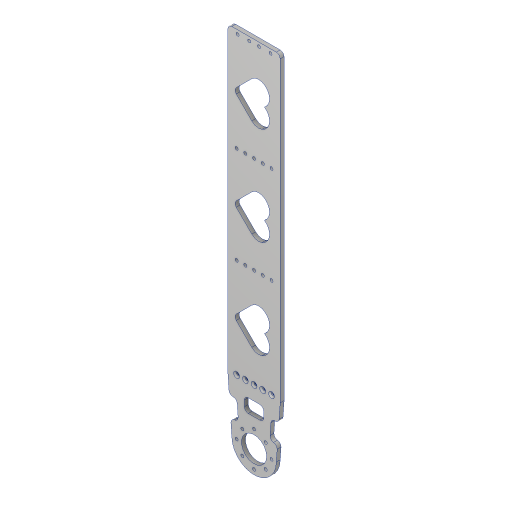
# Autodesk Inventor part: J2L1_H_Side2
Saved by Autodesk Inventor 2023.2 (Build 272271000, 271)
## iProperties
Created: 2021-07-07
Part Number: J2L1_H_Side2
Material: 알루미늄 6061
Document SubType Name: Modeling
Designer: user
Density: 2.7 g/cm^3
Appearance: 알루미늄 - 평지
Mass: 220.087 g
Surface Area: 468.714 cm^2
Volume: 81.5136 cm^3
Author: user
Autodesk Inventor part; units mm, degrees
ref_plane "YZ Plane" through (0, 0, 0) normal (1, 0, 0) x (0, 1, 0)
ref_plane "XZ Plane" through (0, 0, 0) normal (0, 1, 0) x (-1, 0, 0)
ref_plane "XY Plane" through (0, 0, 0) normal (0, 0, 1) x (1, 0, 0)
sketch "스케치1" plane through (0, 0, 0) normal (0, 0, 1) x (1, 0, 0)
  circle A0 centre (0, 0) radius 13
  circle A1 centre (0, 0) radius 23
  line L0 (27, 0) -> (-27, 0)
  line L1 (-27, 0) -> (-27, 62)
  line L2 (-27, 62) -> (27, 62)
  line L3 (27, 62) -> (27, 0)
  line L4 (27, 62) -> (27, 55)
  line L5 (27, 62) -> (34, 62) construction
  line L6 (27, 55) -> (23, 0)
  line L7 (-27, 62) -> (-27, 55)
  line L8 (-27, 62) -> (-20, 62) construction
  line L9 (-27, 55) -> (-23, 0)
  dimension "d0" = 26
  dimension "d1" = 46
  dimension "d2" = 54
  dimension "d3" = 62
  dimension "d4" = 27
  dimension "d5" = 0
  dimension "d6" = 7
  dimension "d7" = 90
  dimension "d8" = 7
  dimension "d9" = 90
  constraints: 20 end point, 3 horizontal, 3 parallel, 3 perpendicular, 2 centre point, 2 coincident, 2 point on circle, 2 point on line, 1 collinear
  measures "d0" diameter of A0
  measures "d1" diameter of A1
  measures "d2" distance of L1.end L2.end
  measures "d3" distance of L0.end L1.end
  measures "d4" distance from line of L3 point (0, 0)
  measures "d5" distance from line of point (0, 0) L0
  measures "d6" distance of L2.end L4.end
  measures "d7" angle of L4 L5
  measures "d8" distance of L1.end L7.end
  measures "d9" angle of L7 L8
extrude "돌출1" add sketch "스케치1" along normal blind 4 contours L0 A0 | L0 A1 A0 | A0 L0 A1 | A0 L0 | A1 L9 L1 L2 L3 L6
sketch "스케치2" plane through (0, 0, 4) normal (0, 0, 1) x (1, 0, 0)
  circle A0 centre (0, 0) radius 13
  dimension "d12" = 26
  constraints: 1 centre point, 1 coincident
  measures "d12" diameter of A0
extrude "돌출2" cut sketch "스케치2" against normal up to surface (4 mm away)
sketch "스케치3" plane through (0, 0, 4) normal (0, 0, 1) x (1, 0, 0)
  line L0 (-0.15, -20.7995) -> (-0.15, -19.593)
  arc A0 (-0.15, -16.407) -> (-0.15, -19.593) centre (0, -18) ccw
  line L1 (-0.15, -16.407) -> (-0.15, -12.9991)
  arc A1 (0.15, -12.9991) -> (-0.15, -12.9991) centre (0, 0) ccw
  line L2 (0.15, -16.407) -> (0.15, -12.9991)
  arc A2 (0.15, -19.593) -> (0.15, -16.407) centre (0, -18) ccw
  line L3 (0.15, -20.7995) -> (0.15, -19.593)
  arc A3 (0.15, -20.7995) -> (-0.15, -20.7995) centre (0, 0) ccw
  circle A4 centre (12, 12) radius 1.6
  circle A5 centre (-18, 0) radius 1.6
  circle A6 centre (-12, 12) radius 1.6
  circle A7 centre (-12, -12) radius 1.6
  circle A8 centre (18, 0) radius 1.6
  circle A9 centre (12, -12) radius 1.6
  circle A10 centre (6, 18) radius 1
  circle A11 centre (-6, 18) radius 1
  circle A12 centre (-18, 6) radius 1
  circle A13 centre (-18, -6) radius 1
  circle A14 centre (-6, -18) radius 1
  circle A15 centre (6, -18) radius 1
  circle A16 centre (18, -6) radius 1
  circle A17 centre (18, 6) radius 1
  circle A18 centre (0, 18) radius 1.6
  circle A19 centre (0, 0) radius 12.5
  line L4 (-27, -21) -> (-21, -21)
  line L5 (-21, -21) -> (-21, -27)
  line L6 (25, -27) -> (27, -25)
  line L7 (27, -25) -> (27, 25)
  line L8 (27, 25) -> (25, 27)
  line L9 (25, 27) -> (-25, 27)
  line L10 (-25, 27) -> (-27, 25)
  line L11 (-27, 25) -> (-27, -25)
  line L12 (-27, -25) -> (-25, -27)
  line L13 (-25, -27) -> (25, -27)
  circle A20 centre (0, 0) radius 26.75
  circle A21 centre (24, -24) radius 1.6
  circle A22 centre (-24, -24) radius 1.6
  circle A23 centre (24, 24) radius 1.6
  circle A24 centre (-24, 24) radius 1.6
  circle A25 centre (0, -18) radius 1.6
  dimension "d15" = 3.2
  constraints: 28 end point, 26 centre point, 8 point on circle, 1 coincident
  measures "d15" diameter of A25
extrude "돌출3" cut sketch "스케치3" against normal up to surface (4 mm away) contours A0 A25 A2 | A4 | A5 | A6 | A7 | A8 | A9 | A18
sketch "스케치4" plane through (0, 0, 4) normal (0, 0, 1) x (1, 0, 0)
  circle A0 centre (0, 18) radius 1.6 projected
  circle A1 centre (12, 12) radius 1.6 projected
  circle A2 centre (-12, 12) radius 1.6 projected
  circle A3 centre (-18, 0) radius 1.6 projected
  circle A4 centre (12, -12) radius 1.6 projected
  circle A5 centre (0, -18) radius 1.6 projected
  circle A6 centre (-12, -12) radius 1.6 projected
  circle A7 centre (18, 0) radius 1.6 projected
  circle A8 centre (0, 0) radius 13 projected
  line L0 (27, 62) -> (-27, 62) projected
  line L1 (-27, 62) -> (-27, 55) projected
  line L2 (-27, 55) -> (-23, 0) projected
  arc A9 (-23, 0) -> (23, 0) centre (0, 0) ccw projected
  line L3 (23, 0) -> (27, 55) projected
  line L4 (27, 55) -> (27, 62) projected
  circle A10 centre (-18, 57.5) radius 1.6
  circle A11 centre (-9, 57.5) radius 1.6
  circle A12 centre (0, 57.5) radius 1.6
  circle A13 centre (9, 57.5) radius 1.6
  circle A14 centre (18, 57.5) radius 1.6
  dimension "d18" = 3.2
  dimension "d19" = 4.5
  dimension "d20" = 3.2
  dimension "d21" = 3.2
  dimension "d22" = 3.2
  dimension "d23" = 3.2
  dimension "d24" = 4.5
  dimension "d25" = 4.5
  dimension "d26" = 4.5
  dimension "d27" = 4.5
  dimension "d28" = 9
  dimension "d29" = 18
  dimension "d30" = 27
  dimension "d31" = 36
  dimension "d32" = 9
  constraints: 5 centre point
  measures "d18" diameter of A10
  measures "d19" distance from line of L0 A10.centre
  measures "d20" diameter of A11
  measures "d21" diameter of A12
  measures "d22" diameter of A13
  measures "d23" diameter of A14
  measures "d24" distance from line of L0 A11.centre
  measures "d25" distance from line of L0 A12.centre
  measures "d26" distance from line of L0 A13.centre
  measures "d27" distance from line of L0 A14.centre
  measures "d28" distance from line of L1 A10.centre
  measures "d29" distance from line of L1 A11.centre
  measures "d30" distance from line of L1 A12.centre
  measures "d31" distance from line of L1 A13.centre
  measures "d32" distance from line of L4 A14.centre
extrude "돌출4" cut sketch "스케치4" against normal up to surface (4 mm away) contours A10 | A11 | A12 | A13 | A14
fillet "모깎기1" radius 5 2 edges at (-27, 62, 2) (27, 62, 2)
sketch "스케치7" plane through (0, 0, 4) normal (0, 0, 1) x (1, 0, 0)
  circle A0 centre (0, 57.5) radius 1.6 projected
  line L0 (0, 0) -> (0, 57.5)
  arc A1 (27, 57) -> (22, 62) centre (22, 57) ccw projected
  line L1 (22, 62) -> (-22, 62) projected
  arc A2 (-22, 62) -> (-27, 57) centre (-22, 57) ccw projected
  line L2 (-27, 57) -> (-27, 55) projected
  line L3 (-27, 55) -> (-23, 0) projected
  arc A3 (-23, 0) -> (23, 0) centre (0, 0) ccw projected
  line L4 (23, 0) -> (27, 55) projected
  line L5 (27, 55) -> (27, 57) projected
  circle A4 centre (9, 57.5) radius 1.6 projected
  circle A5 centre (18, 57.5) radius 1.6 projected
  circle A6 centre (0, 57.5) radius 1.6 projected
  circle A7 centre (-18, 57.5) radius 1.6 projected
  circle A8 centre (-9, 57.5) radius 1.6 projected
  circle A9 centre (0, 18) radius 1.6 projected
  circle A10 centre (12, 12) radius 1.6 projected
  circle A11 centre (-12, 12) radius 1.6 projected
  circle A12 centre (-18, 0) radius 1.6 projected
  circle A13 centre (12, -12) radius 1.6 projected
  circle A14 centre (0, -18) radius 1.6 projected
  circle A15 centre (-12, -12) radius 1.6 projected
  circle A16 centre (18, 0) radius 1.6 projected
  circle A17 centre (0, 0) radius 13 projected
  line L6 (18.9061, 54) -> (14.9978, 0.2596)
  arc A18 (-14.9978, 0.2596) -> (14.9978, 0.2596) centre (0, 0) ccw
  line L7 (-14.9978, 0.2596) -> (-18.9061, 54)
  line L8 (-18.9061, 54) -> (18.9061, 54)
  line L9 (16.1716, 16.4) -> (24.1505, 15.8197)
  line L10 (17.6223, 36.3473) -> (25.6012, 35.767)
  line L11 (-16.1716, 16.4) -> (-24.1505, 15.8197)
  line L12 (-17.6223, 36.3473) -> (-25.6012, 35.767)
  dimension "d43" = 8
  dimension "d44" = 20
  constraints: 16 end point, 4 symmetric about line, 2 point on circle, 2 point on line, 1 centre point, 1 parallel, 1 perpendicular, 3 other
  measures "d43" distance between parallel lines of L4 L6
  measures "d44" distance between parallel lines of L9 L10
extrude "돌출6" cut sketch "스케치7" against normal blind 10 contours L7 L11 L3 L12 | L10 L4 L9 L6
fillet "모깎기3" radius 4 8 edges at (-16.1716, 16.4, 2) (-17.6223, 36.3473, 2) (-25.6012, 35.767, 2) (-24.1505, 15.8197, 2) (25.6012, 35.767, 2) (17.6223, 36.3473, 2) (16.1716, 16.4, 2) (24.1505, 15.8197, 2)
sketch "스케치8" plane through (0, 0, 4) normal (0, 0, 1) x (1, 0, 0)
  line L0 (-10, 43) -> (10, 43)
  line L1 (10, 43) -> (10, 29)
  line L2 (10, 29) -> (-10, 29)
  line L3 (-10, 29) -> (-10, 43)
  point P0 (0, 0)
  dimension "d48" = 14
  dimension "d49" = 20
  dimension "d50" = 10
  constraints: 8 end point, 2 parallel, 1 horizontal, 1 perpendicular
  measures "d48" distance between parallel lines of L2 L0
  measures "d49" distance between parallel lines of L1 L3
  measures "d50" distance from line of L3 point (0, 0)
extrude "돌출7" cut sketch "스케치8" against normal blind 10
fillet "모깎기4" radius 4 4 edges at (-10, 29, 2) (10, 29, 2) (10, 43, 2) (-10, 43, 2)
sketch "스케치9" plane through (0, 0, 4) normal (0, 0, 1) x (1, 0, 0)
  line L0 (10, 39) -> (10, 33) projected
  arc A0 (6, 29) -> (10, 33) centre (6, 33) ccw projected
  line L1 (6, 29) -> (-6, 29) projected
  arc A1 (-10, 33) -> (-6, 29) centre (-6, 33) ccw projected
  line L2 (-10, 33) -> (-10, 39) projected
  arc A2 (-6, 43) -> (-10, 39) centre (-6, 39) ccw projected
  line L3 (-6, 43) -> (6, 43) projected
  arc A3 (10, 39) -> (6, 43) centre (6, 39) ccw projected
  circle A4 centre (0, 0) radius 13 projected
  circle A5 centre (18, 0) radius 1.6 projected
  circle A6 centre (-12, -12) radius 1.6 projected
  circle A7 centre (0, -18) radius 1.6 projected
  circle A8 centre (12, -12) radius 1.6 projected
  circle A9 centre (-18, 0) radius 1.6 projected
  circle A10 centre (-12, 12) radius 1.6 projected
  circle A11 centre (12, 12) radius 1.6 projected
  circle A12 centre (0, 18) radius 1.6 projected
  circle A13 centre (-9, 57.5) radius 1.6 projected
  circle A14 centre (-18, 57.5) radius 1.6 projected
  circle A15 centre (0, 57.5) radius 1.6 projected
  circle A16 centre (18, 57.5) radius 1.6 projected
  circle A17 centre (9, 57.5) radius 1.6 projected
  arc A18 (23.8604, 11.8303) -> (20.1611, 16.1099) centre (19.8709, 12.1204) ccw projected
  arc A19 (16.4617, 20.3895) -> (20.1611, 16.1099) centre (20.4512, 20.0993) ccw projected
  line L4 (16.4617, 20.3895) -> (17.3322, 32.3579) projected
  arc A20 (21.6118, 36.0572) -> (17.3322, 32.3579) centre (21.3216, 32.0677) ccw projected
  arc A21 (21.6118, 36.0572) -> (25.8914, 39.7565) centre (21.9019, 40.0466) ccw projected
  line L5 (25.8914, 39.7565) -> (27, 55) projected
  line L6 (27, 55) -> (27, 57) projected
  arc A22 (27, 57) -> (22, 62) centre (22, 57) ccw projected
  line L7 (22, 62) -> (-22, 62) projected
  arc A23 (-22, 62) -> (-27, 57) centre (-22, 57) ccw projected
  line L8 (-27, 57) -> (-27, 55) projected
  line L9 (-27, 55) -> (-25.8914, 39.7565) projected
  arc A24 (-25.8914, 39.7565) -> (-21.6118, 36.0572) centre (-21.9019, 40.0466) ccw projected
  arc A25 (-17.3322, 32.3579) -> (-21.6118, 36.0572) centre (-21.3216, 32.0677) ccw projected
  line L10 (-17.3322, 32.3579) -> (-16.4617, 20.3895) projected
  arc A26 (-20.1611, 16.1099) -> (-16.4617, 20.3895) centre (-20.4512, 20.0993) ccw projected
  arc A27 (-20.1611, 16.1099) -> (-23.8604, 11.8303) centre (-19.8709, 12.1204) ccw projected
  line L11 (-23.8604, 11.8303) -> (-23, 0) projected
  arc A28 (-23, 0) -> (23, 0) centre (0, 0) ccw projected
  line L12 (23, 0) -> (23.8604, 11.8303) projected
  line L13 (0, 0) -> (0, 420)
  line L14 (0, 210) -> (-51.051, 210)
  line L15 (10, 381) -> (10, 387)
  arc A29 (10, 387) -> (6, 391) centre (6, 387) ccw
  line L16 (6, 391) -> (-6, 391)
  arc A30 (-6, 391) -> (-10, 387) centre (-6, 387) ccw
  line L17 (-10, 387) -> (-10, 381)
  arc A31 (-10, 381) -> (-6, 377) centre (-6, 381) ccw
  line L18 (-6, 377) -> (6, 377)
  arc A32 (6, 377) -> (10, 381) centre (6, 381) ccw
  circle A33 centre (0, 420) radius 13
  circle A34 centre (18, 420) radius 1.6
  circle A35 centre (-12, 432) radius 1.6
  circle A36 centre (0, 438) radius 1.6
  circle A37 centre (12, 432) radius 1.6
  circle A38 centre (-18, 420) radius 1.6
  circle A39 centre (-12, 408) radius 1.6
  circle A40 centre (12, 408) radius 1.6
  circle A41 centre (0, 402) radius 1.6
  circle A42 centre (-9, 362.5) radius 1.6
  circle A43 centre (-18, 362.5) radius 1.6
  circle A44 centre (0, 362.5) radius 1.6
  circle A45 centre (18, 362.5) radius 1.6
  circle A46 centre (9, 362.5) radius 1.6
  arc A47 (20.1611, 403.8901) -> (23.8604, 408.1697) centre (19.8709, 407.8796) ccw
  arc A48 (20.1611, 403.8901) -> (16.4617, 399.6105) centre (20.4512, 399.9007) ccw
  line L19 (16.4617, 399.6105) -> (17.3322, 387.6421)
  arc A49 (17.3322, 387.6421) -> (21.6118, 383.9428) centre (21.3216, 387.9323) ccw
  arc A50 (25.8914, 380.2435) -> (21.6118, 383.9428) centre (21.9019, 379.9534) ccw
  line L20 (25.8914, 380.2435) -> (27, 365)
  line L21 (27, 365) -> (27, 363)
  arc A51 (22, 358) -> (27, 363) centre (22, 363) ccw
  line L22 (22, 358) -> (-22, 358)
  arc A52 (-27, 363) -> (-22, 358) centre (-22, 363) ccw
  line L23 (-27, 363) -> (-27, 365)
  line L24 (-27, 365) -> (-25.8914, 380.2435)
  arc A53 (-21.6118, 383.9428) -> (-25.8914, 380.2435) centre (-21.9019, 379.9534) ccw
  arc A54 (-21.6118, 383.9428) -> (-17.3322, 387.6421) centre (-21.3216, 387.9323) ccw
  line L25 (-17.3322, 387.6421) -> (-16.4617, 399.6105)
  arc A55 (-16.4617, 399.6105) -> (-20.1611, 403.8901) centre (-20.4512, 399.9007) ccw
  arc A56 (-23.8604, 408.1697) -> (-20.1611, 403.8901) centre (-19.8709, 407.8796) ccw
  line L26 (-23.8604, 408.1697) -> (-23, 420)
  arc A57 (23, 420) -> (-23, 420) centre (0, 420) ccw
  line L27 (23, 420) -> (23.8604, 408.1697)
  line L28 (-27, 57) -> (-27, 55) projected
  line L29 (-27, 57) -> (-27, 363)
  arc A58 (27, 57) -> (22, 62) centre (22, 57) ccw projected
  line L30 (27, 57) -> (27, 363)
  dimension "d54" = 420
  constraints: 57 symmetric about line, 34 end point, 30 point on circle, 29 centre point, 1 collinear, 1 horizontal, 1 midpoint, 1 parallel, 1 tangent, 1 vertical, 29 other
  measures "d54" distance of L13.start L13.end
extrude "돌출8" add sketch "스케치9" against normal blind 4 contours L7 A23 L29 L14 L13 | L13 L22 A51 L30 A22 L7 | L14 L29 A52 L22 L13 | L22 A52 L23 L24 A53 A54 L25 A55 A56 L26 A57 L27 A47 A48 L19 A49 A50 L20 L21 A51
sketch "스케치10" plane through (0, 0, 4) normal (0, 0, 1) x (1, 0, 0)
  line L0 (-27, 365) -> (-25.8914, 380.2435) projected
  line L1 (-26.4457, 372.6218) -> (26.4457, 372.6218)
  line L2 (27, 365) -> (25.8914, 380.2435) projected
  circle A0 centre (0, 362.5) radius 1.6 projected
  circle A1 centre (-12, 408) radius 1.6 projected
  circle A2 centre (18, 420) radius 1.6 projected
  circle A3 centre (-12, 432) radius 1.6 projected
  circle A4 centre (0, 438) radius 1.6 projected
  circle A5 centre (12, 432) radius 1.6 projected
  circle A6 centre (12, 408) radius 1.6 projected
  circle A7 centre (-18, 420) radius 1.6 projected
  circle A8 centre (-18, 362.5) radius 1.6 projected
  circle A9 centre (9, 362.5) radius 1.6 projected
  circle A10 centre (18, 362.5) radius 1.6 projected
  circle A11 centre (-9, 362.5) radius 1.6 projected
  line L3 (-6, 391) -> (6, 391) projected
  arc A12 (10, 387) -> (6, 391) centre (6, 387) ccw projected
  line L4 (10, 387) -> (10, 381) projected
  arc A13 (6, 377) -> (10, 381) centre (6, 381) ccw projected
  line L5 (6, 377) -> (-6, 377) projected
  arc A14 (-10, 381) -> (-6, 377) centre (-6, 381) ccw projected
  line L6 (-10, 381) -> (-10, 387) projected
  arc A15 (-6, 391) -> (-10, 387) centre (-6, 387) ccw projected
  circle A16 centre (0, 402) radius 1.6 projected
  circle A17 centre (0, 420) radius 13 projected
  line L7 (10, 39) -> (10, 33) projected
  arc A18 (6, 29) -> (10, 33) centre (6, 33) ccw projected
  line L8 (6, 29) -> (-6, 29) projected
  arc A19 (-10, 33) -> (-6, 29) centre (-6, 33) ccw projected
  line L9 (-10, 33) -> (-10, 39) projected
  arc A20 (-6, 43) -> (-10, 39) centre (-6, 39) ccw projected
  line L10 (-6, 43) -> (6, 43) projected
  arc A21 (10, 39) -> (6, 43) centre (6, 39) ccw projected
  circle A22 centre (0, 0) radius 13 projected
  circle A23 centre (18, 0) radius 1.6 projected
  circle A24 centre (-12, -12) radius 1.6 projected
  circle A25 centre (0, -18) radius 1.6 projected
  circle A26 centre (12, -12) radius 1.6 projected
  circle A27 centre (-18, 0) radius 1.6 projected
  circle A28 centre (-12, 12) radius 1.6 projected
  circle A29 centre (12, 12) radius 1.6 projected
  circle A30 centre (0, 18) radius 1.6 projected
  circle A31 centre (-9, 57.5) radius 1.6 projected
  circle A32 centre (-18, 57.5) radius 1.6 projected
  circle A33 centre (0, 57.5) radius 1.6 projected
  circle A34 centre (18, 57.5) radius 1.6 projected
  circle A35 centre (9, 57.5) radius 1.6 projected
  arc A36 (23.8604, 11.8303) -> (20.1611, 16.1099) centre (19.8709, 12.1204) ccw projected
  arc A37 (16.4617, 20.3895) -> (20.1611, 16.1099) centre (20.4512, 20.0993) ccw projected
  line L11 (16.4617, 20.3895) -> (17.3322, 32.3579) projected
  arc A38 (21.6118, 36.0572) -> (17.3322, 32.3579) centre (21.3216, 32.0677) ccw projected
  arc A39 (21.6118, 36.0572) -> (25.8914, 39.7565) centre (21.9019, 40.0466) ccw projected
  line L12 (25.8914, 39.7565) -> (27, 55) projected
  line L13 (27, 55) -> (27, 365) projected
  line L14 (27, 365) -> (25.8914, 380.2435) projected
  arc A40 (25.8914, 380.2435) -> (21.6118, 383.9428) centre (21.9019, 379.9534) ccw projected
  arc A41 (17.3322, 387.6421) -> (21.6118, 383.9428) centre (21.3216, 387.9323) ccw projected
  line L15 (17.3322, 387.6421) -> (16.4617, 399.6105) projected
  arc A42 (20.1611, 403.8901) -> (16.4617, 399.6105) centre (20.4512, 399.9007) ccw projected
  arc A43 (20.1611, 403.8901) -> (23.8604, 408.1697) centre (19.8709, 407.8796) ccw projected
  line L16 (23.8604, 408.1697) -> (23, 420) projected
  arc A44 (23, 420) -> (-23, 420) centre (0, 420) ccw projected
  line L17 (-23, 420) -> (-23.8604, 408.1697) projected
  arc A45 (-23.8604, 408.1697) -> (-20.1611, 403.8901) centre (-19.8709, 407.8796) ccw projected
  arc A46 (-16.4617, 399.6105) -> (-20.1611, 403.8901) centre (-20.4512, 399.9007) ccw projected
  line L18 (-16.4617, 399.6105) -> (-17.3322, 387.6421) projected
  arc A47 (-21.6118, 383.9428) -> (-17.3322, 387.6421) centre (-21.3216, 387.9323) ccw projected
  arc A48 (-21.6118, 383.9428) -> (-25.8914, 380.2435) centre (-21.9019, 379.9534) ccw projected
  line L19 (-25.8914, 380.2435) -> (-27, 365) projected
  line L20 (-27, 365) -> (-27, 55) projected
  line L21 (-27, 55) -> (-25.8914, 39.7565) projected
  arc A49 (-25.8914, 39.7565) -> (-21.6118, 36.0572) centre (-21.9019, 40.0466) ccw projected
  arc A50 (-17.3322, 32.3579) -> (-21.6118, 36.0572) centre (-21.3216, 32.0677) ccw projected
  line L22 (-17.3322, 32.3579) -> (-16.4617, 20.3895) projected
  arc A51 (-20.1611, 16.1099) -> (-16.4617, 20.3895) centre (-20.4512, 20.0993) ccw projected
  arc A52 (-20.1611, 16.1099) -> (-23.8604, 11.8303) centre (-19.8709, 12.1204) ccw projected
  line L23 (-23.8604, 11.8303) -> (-23, 0) projected
  arc A53 (-23, 0) -> (23, 0) centre (0, 0) ccw projected
  line L24 (23, 0) -> (23.8604, 11.8303) projected
  point P0 (25.8914, 380.2435)
  point P1 (-25.8914, 380.2435)
  constraints: 2 end point, 2 midpoint
extrude "돌출9" cut sketch "스케치10" against normal blind 4 contours L0 A48 A47 L18 A46 A45 L17 A44 L16 A43 A42 L15 A41 A40 L2 L1
fillet "모깎기5" radius 2 2 edges at (-26.4457, 372.6218, 2) (26.4457, 372.6218, 2)
sketch "스케치11" plane through (0, 0, 4) normal (0, 0, 1) x (1, 0, 0)
  arc A0 (26.5806, 370.7668) -> (24.5859, 372.6218) centre (24.5859, 370.6218) ccw projected
  line L0 (24.5859, 372.6218) -> (-24.5859, 372.6218) projected
  arc A1 (-24.5859, 372.6218) -> (-26.5806, 370.7668) centre (-24.5859, 370.6218) ccw projected
  line L1 (-26.5806, 370.7668) -> (-27, 365) projected
  line L2 (-27, 365) -> (-27, 55) projected
  line L3 (-27, 55) -> (-25.8914, 39.7565) projected
  arc A2 (-25.8914, 39.7565) -> (-21.6118, 36.0572) centre (-21.9019, 40.0466) ccw projected
  arc A3 (-17.3322, 32.3579) -> (-21.6118, 36.0572) centre (-21.3216, 32.0677) ccw projected
  line L4 (-17.3322, 32.3579) -> (-16.4617, 20.3895) projected
  arc A4 (-20.1611, 16.1099) -> (-16.4617, 20.3895) centre (-20.4512, 20.0993) ccw projected
  arc A5 (-20.1611, 16.1099) -> (-23.8604, 11.8303) centre (-19.8709, 12.1204) ccw projected
  line L5 (-23.8604, 11.8303) -> (-23, 0) projected
  arc A6 (-23, 0) -> (23, 0) centre (0, 0) ccw projected
  line L6 (23, 0) -> (23.8604, 11.8303) projected
  arc A7 (23.8604, 11.8303) -> (20.1611, 16.1099) centre (19.8709, 12.1204) ccw projected
  arc A8 (16.4617, 20.3895) -> (20.1611, 16.1099) centre (20.4512, 20.0993) ccw projected
  line L7 (16.4617, 20.3895) -> (17.3322, 32.3579) projected
  arc A9 (21.6118, 36.0572) -> (17.3322, 32.3579) centre (21.3216, 32.0677) ccw projected
  arc A10 (21.6118, 36.0572) -> (25.8914, 39.7565) centre (21.9019, 40.0466) ccw projected
  line L8 (25.8914, 39.7565) -> (27, 55) projected
  line L9 (27, 55) -> (27, 365) projected
  line L10 (27, 365) -> (26.5806, 370.7668) projected
  circle A11 centre (0, 362.5) radius 1.6 projected
  circle A12 centre (-18, 362.5) radius 1.6 projected
  circle A13 centre (9, 362.5) radius 1.6 projected
  circle A14 centre (18, 362.5) radius 1.6 projected
  circle A15 centre (-9, 362.5) radius 1.6 projected
  line L11 (10, 39) -> (10, 33) projected
  arc A16 (6, 29) -> (10, 33) centre (6, 33) ccw projected
  line L12 (6, 29) -> (-6, 29) projected
  arc A17 (-10, 33) -> (-6, 29) centre (-6, 33) ccw projected
  line L13 (-10, 33) -> (-10, 39) projected
  arc A18 (-6, 43) -> (-10, 39) centre (-6, 39) ccw projected
  line L14 (-6, 43) -> (6, 43) projected
  arc A19 (10, 39) -> (6, 43) centre (6, 39) ccw projected
  circle A20 centre (0, 0) radius 13 projected
  circle A21 centre (18, 0) radius 1.6 projected
  circle A22 centre (-12, -12) radius 1.6 projected
  circle A23 centre (0, -18) radius 1.6 projected
  circle A24 centre (12, -12) radius 1.6 projected
  circle A25 centre (-18, 0) radius 1.6 projected
  circle A26 centre (-12, 12) radius 1.6 projected
  circle A27 centre (12, 12) radius 1.6 projected
  circle A28 centre (0, 18) radius 1.6 projected
  circle A29 centre (-9, 57.5) radius 1.6 projected
  circle A30 centre (-18, 57.5) radius 1.6 projected
  circle A31 centre (0, 57.5) radius 1.6 projected
  circle A32 centre (18, 57.5) radius 1.6 projected
  circle A33 centre (9, 57.5) radius 1.6 projected
  circle A34 centre (18, 57.5) radius 1.6 projected
  circle A35 centre (9, 57.5) radius 1.6 projected
  circle A36 centre (0, 57.5) radius 1.6 projected
  circle A37 centre (-9, 57.5) radius 1.6 projected
  circle A38 centre (-18, 57.5) radius 1.6 projected
  line L15 (-27, 365) -> (-27, 55) projected
  line L16 (-27, 365) -> (-27, 55) projected
  circle A39 centre (18, 57.5) radius 1.6 projected
  circle A40 centre (9, 57.5) radius 1.6 projected
  circle A41 centre (0, 57.5) radius 1.6 projected
  circle A42 centre (-9, 57.5) radius 1.6 projected
  circle A43 centre (-18, 57.5) radius 1.6 projected
  circle A44 centre (-18, 362.5) radius 1.6 projected
  line L17 (-18, 57.5) -> (-18, 362.5) construction
  circle A45 centre (-9, 362.5) radius 1.6 projected
  line L18 (-9, 57.5) -> (-9, 362.5) construction
  circle A46 centre (-18, 210) radius 1.6
  circle A47 centre (-18, 160) radius 1.6
  circle A48 centre (-18, 260) radius 1.6
  circle A49 centre (-9, 160) radius 1.6
  circle A50 centre (-9, 210) radius 1.6
  circle A51 centre (-9, 260) radius 1.6
  line L19 (0, 0) -> (0, 362.5)
  circle A52 centre (18, 210) radius 1.6
  circle A53 centre (18, 160) radius 1.6
  circle A54 centre (18, 260) radius 1.6
  circle A55 centre (9, 160) radius 1.6
  circle A56 centre (9, 210) radius 1.6
  circle A57 centre (9, 260) radius 1.6
  dimension "d60" = 3.2
  dimension "d61" = 50
  dimension "d62" = 50
  constraints: 12 centre point, 6 end point, 6 symmetric about line, 5 equal radius, 4 point on line, 3 horizontal alignment, 3 vertical, 2 midpoint, 6 other
  measures "d60" diameter of A50
  measures "d61" distance of A46.centre A48.centre
  measures "d62" distance of A47.centre A46.centre
extrude "돌출10" cut sketch "스케치11" against normal blind 4 contours A46 | A47 | A48 | A49 | A50 | A51 | A52 | A53 | A54 | A55 | A56 | A57
sketch "스케치12" plane through (0, 0, 4) normal (0, 0, 1) x (1, 0, 0)
  circle A0 centre (9, 160) radius 1.6 projected
  circle A1 centre (9, 210) radius 1.6 projected
  circle A2 centre (9, 260) radius 1.6 projected
  circle A3 centre (-9, 260) radius 1.6 projected
  circle A4 centre (-9, 210) radius 1.6 projected
  circle A5 centre (-9, 160) radius 1.6 projected
  circle A6 centre (18, 160) radius 1.6 projected
  circle A7 centre (18, 210) radius 1.6 projected
  circle A8 centre (18, 260) radius 1.6 projected
  circle A9 centre (-18, 260) radius 1.6 projected
  circle A10 centre (-18, 210) radius 1.6 projected
  circle A11 centre (-18, 160) radius 1.6 projected
  arc A12 (26.5806, 370.7668) -> (24.5859, 372.6218) centre (24.5859, 370.6218) ccw projected
  line L0 (24.5859, 372.6218) -> (-24.5859, 372.6218) projected
  arc A13 (-24.5859, 372.6218) -> (-26.5806, 370.7668) centre (-24.5859, 370.6218) ccw projected
  line L1 (-26.5806, 370.7668) -> (-27, 365) projected
  line L2 (-27, 365) -> (-27, 55) projected
  line L3 (-27, 55) -> (-25.8914, 39.7565) projected
  arc A14 (-25.8914, 39.7565) -> (-21.6118, 36.0572) centre (-21.9019, 40.0466) ccw projected
  arc A15 (-17.3322, 32.3579) -> (-21.6118, 36.0572) centre (-21.3216, 32.0677) ccw projected
  line L4 (-17.3322, 32.3579) -> (-16.4617, 20.3895) projected
  arc A16 (-20.1611, 16.1099) -> (-16.4617, 20.3895) centre (-20.4512, 20.0993) ccw projected
  arc A17 (-20.1611, 16.1099) -> (-23.8604, 11.8303) centre (-19.8709, 12.1204) ccw projected
  line L5 (-23.8604, 11.8303) -> (-23, 0) projected
  arc A18 (-23, 0) -> (23, 0) centre (0, 0) ccw projected
  line L6 (23, 0) -> (23.8604, 11.8303) projected
  arc A19 (23.8604, 11.8303) -> (20.1611, 16.1099) centre (19.8709, 12.1204) ccw projected
  arc A20 (16.4617, 20.3895) -> (20.1611, 16.1099) centre (20.4512, 20.0993) ccw projected
  line L7 (16.4617, 20.3895) -> (17.3322, 32.3579) projected
  arc A21 (21.6118, 36.0572) -> (17.3322, 32.3579) centre (21.3216, 32.0677) ccw projected
  arc A22 (21.6118, 36.0572) -> (25.8914, 39.7565) centre (21.9019, 40.0466) ccw projected
  line L8 (25.8914, 39.7565) -> (27, 55) projected
  line L9 (27, 55) -> (27, 365) projected
  line L10 (27, 365) -> (26.5806, 370.7668) projected
  circle A23 centre (0, 362.5) radius 1.6 projected
  circle A24 centre (-18, 362.5) radius 1.6 projected
  circle A25 centre (9, 362.5) radius 1.6 projected
  circle A26 centre (18, 362.5) radius 1.6 projected
  circle A27 centre (-9, 362.5) radius 1.6 projected
  line L11 (10, 39) -> (10, 33) projected
  arc A28 (6, 29) -> (10, 33) centre (6, 33) ccw projected
  line L12 (6, 29) -> (-6, 29) projected
  arc A29 (-10, 33) -> (-6, 29) centre (-6, 33) ccw projected
  line L13 (-10, 33) -> (-10, 39) projected
  arc A30 (-6, 43) -> (-10, 39) centre (-6, 39) ccw projected
  line L14 (-6, 43) -> (6, 43) projected
  arc A31 (10, 39) -> (6, 43) centre (6, 39) ccw projected
  circle A32 centre (0, 0) radius 13 projected
  circle A33 centre (18, 0) radius 1.6 projected
  circle A34 centre (-12, -12) radius 1.6 projected
  circle A35 centre (0, -18) radius 1.6 projected
  circle A36 centre (12, -12) radius 1.6 projected
  circle A37 centre (-18, 0) radius 1.6 projected
  circle A38 centre (-12, 12) radius 1.6 projected
  circle A39 centre (12, 12) radius 1.6 projected
  circle A40 centre (0, 18) radius 1.6 projected
  circle A41 centre (-9, 57.5) radius 1.6 projected
  circle A42 centre (-18, 57.5) radius 1.6 projected
  circle A43 centre (0, 57.5) radius 1.6 projected
  circle A44 centre (18, 57.5) radius 1.6 projected
  circle A45 centre (9, 57.5) radius 1.6 projected
  line L15 (-27, 365) -> (-27, 55) projected
  line L16 (-27, 362.5) -> (0, 362.5)
  line L17 (-27, 365) -> (-27, 372.6218)
  line L18 (-27, 372.6218) -> (27, 372.6218)
  line L19 (27, 372.6218) -> (27, 365)
  circle A46 centre (0, 362.5) radius 1.6 projected
  line L20 (0, 362.5) -> (0, 366.5)
  line L21 (0, 366.5) -> (-27, 366.5)
  line L22 (0, 366.5) -> (27, 366.5)
  point P0 (26.8909, 366.5)
  point P1 (-26.8909, 366.5)
  dimension "d65" = 4
  constraints: 14 end point, 6 point on line, 3 perpendicular, 1 vertical
  measures "d65" distance of L20.start L20.end
extrude "돌출11" cut sketch "스케치12" against normal blind 4 contours L10 L22 L21 L1 A13 L0 A12
sketch "스케치13" plane through (0, 0, 4) normal (0, 0, 1) x (1, 0, 0)
  line L0 (26.8909, 366.5) -> (-26.8909, 366.5) projected
  line L1 (-26.8909, 366.5) -> (-27, 365) projected
  line L2 (-27, 365) -> (-27, 55) projected
  line L3 (-27, 55) -> (-25.8914, 39.7565) projected
  arc A0 (-25.8914, 39.7565) -> (-21.6118, 36.0572) centre (-21.9019, 40.0466) ccw projected
  arc A1 (-17.3322, 32.3579) -> (-21.6118, 36.0572) centre (-21.3216, 32.0677) ccw projected
  line L4 (-17.3322, 32.3579) -> (-16.4617, 20.3895) projected
  arc A2 (-20.1611, 16.1099) -> (-16.4617, 20.3895) centre (-20.4512, 20.0993) ccw projected
  arc A3 (-20.1611, 16.1099) -> (-23.8604, 11.8303) centre (-19.8709, 12.1204) ccw projected
  line L5 (-23.8604, 11.8303) -> (-23, 0) projected
  arc A4 (-23, 0) -> (23, 0) centre (0, 0) ccw projected
  line L6 (23, 0) -> (23.8604, 11.8303) projected
  arc A5 (23.8604, 11.8303) -> (20.1611, 16.1099) centre (19.8709, 12.1204) ccw projected
  arc A6 (16.4617, 20.3895) -> (20.1611, 16.1099) centre (20.4512, 20.0993) ccw projected
  line L7 (16.4617, 20.3895) -> (17.3322, 32.3579) projected
  arc A7 (21.6118, 36.0572) -> (17.3322, 32.3579) centre (21.3216, 32.0677) ccw projected
  arc A8 (21.6118, 36.0572) -> (25.8914, 39.7565) centre (21.9019, 40.0466) ccw projected
  line L8 (25.8914, 39.7565) -> (27, 55) projected
  line L9 (27, 55) -> (27, 365) projected
  line L10 (27, 365) -> (26.8909, 366.5) projected
  circle A9 centre (9, 160) radius 1.6 projected
  circle A10 centre (9, 210) radius 1.6 projected
  circle A11 centre (9, 260) radius 1.6 projected
  circle A12 centre (-9, 260) radius 1.6 projected
  circle A13 centre (-9, 210) radius 1.6 projected
  circle A14 centre (-9, 160) radius 1.6 projected
  circle A15 centre (18, 160) radius 1.6 projected
  circle A16 centre (18, 210) radius 1.6 projected
  circle A17 centre (18, 260) radius 1.6 projected
  circle A18 centre (-18, 260) radius 1.6 projected
  circle A19 centre (-18, 210) radius 1.6 projected
  circle A20 centre (-18, 160) radius 1.6 projected
  circle A21 centre (0, 362.5) radius 1.6 projected
  circle A22 centre (-18, 362.5) radius 1.6 projected
  circle A23 centre (9, 362.5) radius 1.6 projected
  circle A24 centre (18, 362.5) radius 1.6 projected
  circle A25 centre (-9, 362.5) radius 1.6 projected
  line L11 (10, 39) -> (10, 33) projected
  arc A26 (6, 29) -> (10, 33) centre (6, 33) ccw projected
  line L12 (6, 29) -> (-6, 29) projected
  arc A27 (-10, 33) -> (-6, 29) centre (-6, 33) ccw projected
  line L13 (-10, 33) -> (-10, 39) projected
  arc A28 (-6, 43) -> (-10, 39) centre (-6, 39) ccw projected
  line L14 (-6, 43) -> (6, 43) projected
  arc A29 (10, 39) -> (6, 43) centre (6, 39) ccw projected
  circle A30 centre (0, 0) radius 13 projected
  circle A31 centre (18, 0) radius 1.6 projected
  circle A32 centre (-12, -12) radius 1.6 projected
  circle A33 centre (0, -18) radius 1.6 projected
  circle A34 centre (12, -12) radius 1.6 projected
  circle A35 centre (-18, 0) radius 1.6 projected
  circle A36 centre (-12, 12) radius 1.6 projected
  circle A37 centre (12, 12) radius 1.6 projected
  circle A38 centre (0, 18) radius 1.6 projected
  circle A39 centre (-9, 57.5) radius 1.6 projected
  circle A40 centre (-18, 57.5) radius 1.6 projected
  circle A41 centre (0, 57.5) radius 1.6 projected
  circle A42 centre (18, 57.5) radius 1.6 projected
  circle A43 centre (9, 57.5) radius 1.6 projected
extrude "돌출12" add sketch "스케치13" against normal blind 4 contours A10 | A13 | A16 | A19
extrude "돌출13" add sketch "스케치12" against normal blind 4 contours L22 L19 L10 | L1 L17 L21
fillet "모깎기6" radius 4 2 edges at (-27, 366.5, 2) (27, 366.5, 2)
sketch "스케치14" plane through (0, 0, 4) normal (0, 0, 1) x (1, 0, 0)
  arc A0 (27, 362.5) -> (23, 366.5) centre (23, 362.5) ccw projected
  line L0 (23, 366.5) -> (-23, 366.5) projected
  arc A1 (-23, 366.5) -> (-27, 362.5) centre (-23, 362.5) ccw projected
  line L1 (-27, 362.5) -> (-27, 55) projected
  line L2 (-27, 55) -> (-25.8914, 39.7565) projected
  arc A2 (-25.8914, 39.7565) -> (-21.6118, 36.0572) centre (-21.9019, 40.0466) ccw projected
  arc A3 (-17.3322, 32.3579) -> (-21.6118, 36.0572) centre (-21.3216, 32.0677) ccw projected
  line L3 (-17.3322, 32.3579) -> (-16.4617, 20.3895) projected
  arc A4 (-20.1611, 16.1099) -> (-16.4617, 20.3895) centre (-20.4512, 20.0993) ccw projected
  arc A5 (-20.1611, 16.1099) -> (-23.8604, 11.8303) centre (-19.8709, 12.1204) ccw projected
  line L4 (-23.8604, 11.8303) -> (-23, 0) projected
  arc A6 (-23, 0) -> (23, 0) centre (0, 0) ccw projected
  line L5 (23, 0) -> (23.8604, 11.8303) projected
  arc A7 (23.8604, 11.8303) -> (20.1611, 16.1099) centre (19.8709, 12.1204) ccw projected
  arc A8 (16.4617, 20.3895) -> (20.1611, 16.1099) centre (20.4512, 20.0993) ccw projected
  line L6 (16.4617, 20.3895) -> (17.3322, 32.3579) projected
  arc A9 (21.6118, 36.0572) -> (17.3322, 32.3579) centre (21.3216, 32.0677) ccw projected
  arc A10 (21.6118, 36.0572) -> (25.8914, 39.7565) centre (21.9019, 40.0466) ccw projected
  line L7 (25.8914, 39.7565) -> (27, 55) projected
  line L8 (27, 55) -> (27, 362.5) projected
  circle A11 centre (9, 160) radius 1.6 projected
  circle A12 centre (9, 260) radius 1.6 projected
  circle A13 centre (-9, 260) radius 1.6 projected
  circle A14 centre (-9, 160) radius 1.6 projected
  circle A15 centre (18, 160) radius 1.6 projected
  circle A16 centre (18, 260) radius 1.6 projected
  circle A17 centre (-18, 260) radius 1.6 projected
  circle A18 centre (-18, 160) radius 1.6 projected
  circle A19 centre (0, 362.5) radius 1.6 projected
  circle A20 centre (-18, 362.5) radius 1.6 projected
  circle A21 centre (9, 362.5) radius 1.6 projected
  circle A22 centre (18, 362.5) radius 1.6 projected
  circle A23 centre (-9, 362.5) radius 1.6 projected
  line L9 (10, 39) -> (10, 33) projected
  arc A24 (6, 29) -> (10, 33) centre (6, 33) ccw projected
  line L10 (6, 29) -> (-6, 29) projected
  arc A25 (-10, 33) -> (-6, 29) centre (-6, 33) ccw projected
  line L11 (-10, 33) -> (-10, 39) projected
  arc A26 (-6, 43) -> (-10, 39) centre (-6, 39) ccw projected
  line L12 (-6, 43) -> (6, 43) projected
  arc A27 (10, 39) -> (6, 43) centre (6, 39) ccw projected
  circle A28 centre (0, 0) radius 13 projected
  circle A29 centre (18, 0) radius 1.6 projected
  circle A30 centre (-12, -12) radius 1.6 projected
  circle A31 centre (0, -18) radius 1.6 projected
  circle A32 centre (12, -12) radius 1.6 projected
  circle A33 centre (-18, 0) radius 1.6 projected
  circle A34 centre (-12, 12) radius 1.6 projected
  circle A35 centre (12, 12) radius 1.6 projected
  circle A36 centre (0, 18) radius 1.6 projected
  circle A37 centre (-9, 57.5) radius 1.6 projected
  circle A38 centre (-18, 57.5) radius 1.6 projected
  circle A39 centre (0, 57.5) radius 1.6 projected
  circle A40 centre (18, 57.5) radius 1.6 projected
  circle A41 centre (9, 57.5) radius 1.6 projected
  circle A42 centre (0, 160) radius 1.6
  circle A43 centre (0, 260) radius 1.6
  circle A44 centre (0, 57.5) radius 1.6 projected
  line L13 (0, 57.5) -> (0, 160) construction
  line L14 (-15, 78.75) -> (15, 78.75)
  line L15 (15, 78.75) -> (15, 138.75)
  line L16 (15, 138.75) -> (-15, 138.75)
  line L17 (-15, 138.75) -> (-15, 78.75)
  line L18 (-15, 78.75) -> (15, 138.75) construction
  line L19 (15, 78.75) -> (-15, 138.75) construction
  circle A45 centre (0, 362.5) radius 1.6 projected
  line L20 (0, 160) -> (0, 362.5) construction
  line L21 (-15, 180) -> (15, 180)
  line L22 (15, 180) -> (15, 240)
  line L23 (15, 240) -> (-15, 240)
  line L24 (-15, 240) -> (-15, 180)
  line L25 (-15, 180) -> (15, 240) construction
  line L26 (15, 180) -> (-15, 240) construction
  line L27 (-15, 281.25) -> (15, 281.25)
  line L28 (15, 281.25) -> (15, 341.25)
  line L29 (15, 341.25) -> (-15, 341.25)
  line L30 (-15, 341.25) -> (-15, 281.25)
  line L31 (-15, 281.25) -> (15, 341.25) construction
  line L32 (15, 281.25) -> (-15, 341.25) construction
  line L33 (-15, 78.75) -> (0, 108.75)
  line L34 (-15, 138.75) -> (0, 108.75)
  line L35 (0, 108.75) -> (15, 138.75)
  line L36 (0, 108.75) -> (15, 78.75)
  circle A46 centre (0, 108.75) radius 5
  line L37 (-15, 180) -> (15, 240)
  line L38 (-15, 240) -> (15, 180)
  line L39 (-15, 281.25) -> (15, 341.25)
  line L40 (-15, 341.25) -> (15, 281.25)
  circle A47 centre (0, 210) radius 5
  circle A48 centre (0, 311.25) radius 5
  point P0 (-2.2361, 113.2221)
  point P1 (2.2361, 113.2221)
  point P2 (2.2361, 104.2779)
  point P3 (-2.2361, 104.2779)
  point P4 (-2.2361, 315.7221)
  point P5 (2.2361, 315.7221)
  point P6 (2.2361, 306.7779)
  point P7 (-2.2361, 306.7779)
  point P8 (-2.2361, 214.4721)
  point P9 (2.2361, 214.4721)
  point P10 (2.2361, 205.5279)
  point P11 (-2.2361, 205.5279)
  dimension "d73" = 3.2
  dimension "d74" = 3.2
  dimension "d75" = 30
  dimension "d76" = 60
  dimension "d77" = 30
  dimension "d78" = 60
  dimension "d79" = 20
  dimension "d80" = 30
  dimension "d81" = 60
  dimension "d82" = 51.25
  dimension "d99" = 21.25
  dimension "d100" = 10
  dimension "d103" = 10
  dimension "d104" = 10
  constraints: 56 end point, 7 midpoint, 6 parallel, 5 centre point, 5 collinear, 3 coincident, 3 horizontal, 3 perpendicular, 2 point on line, 2 vertical, 1 horizontal alignment
  measures "d73" diameter of A42
  measures "d74" diameter of A43
  measures "d75" distance of L16.end L15.end
  measures "d76" distance of L15.end L14.end
  measures "d77" distance of L23.end L22.end
  measures "d78" distance of L22.end L21.end
  measures "d79" distance from line of L23 A43.centre
  measures "d80" distance of L29.end L28.end
  measures "d81" distance of L28.end L27.end
  measures "d82" distance of A19.centre point (0, 311.25)
  measures "d99" distance from line of A39.centre L14
  measures "d100" diameter of A46
  measures "d103" diameter of A47
  measures "d104" diameter of A48
extrude "돌출15" cut sketch "스케치14" against normal blind 4 contours A42 | A43
sketch "스케치15" plane through (0, 0, 4) normal (0, 0, 1) x (1, 0, 0)
  circle A0 centre (0, 260) radius 1.6 projected
  circle A1 centre (0, 160) radius 1.6 projected
  arc A2 (27, 362.5) -> (23, 366.5) centre (23, 362.5) ccw projected
  line L0 (23, 366.5) -> (-23, 366.5) projected
  arc A3 (-23, 366.5) -> (-27, 362.5) centre (-23, 362.5) ccw projected
  line L1 (-27, 362.5) -> (-27, 55) projected
  line L2 (-27, 55) -> (-25.8914, 39.7565) projected
  arc A4 (-25.8914, 39.7565) -> (-21.6118, 36.0572) centre (-21.9019, 40.0466) ccw projected
  arc A5 (-17.3322, 32.3579) -> (-21.6118, 36.0572) centre (-21.3216, 32.0677) ccw projected
  line L3 (-17.3322, 32.3579) -> (-16.4617, 20.3895) projected
  arc A6 (-20.1611, 16.1099) -> (-16.4617, 20.3895) centre (-20.4512, 20.0993) ccw projected
  arc A7 (-20.1611, 16.1099) -> (-23.8604, 11.8303) centre (-19.8709, 12.1204) ccw projected
  line L4 (-23.8604, 11.8303) -> (-23, 0) projected
  arc A8 (-23, 0) -> (23, 0) centre (0, 0) ccw projected
  line L5 (23, 0) -> (23.8604, 11.8303) projected
  arc A9 (23.8604, 11.8303) -> (20.1611, 16.1099) centre (19.8709, 12.1204) ccw projected
  arc A10 (16.4617, 20.3895) -> (20.1611, 16.1099) centre (20.4512, 20.0993) ccw projected
  line L6 (16.4617, 20.3895) -> (17.3322, 32.3579) projected
  arc A11 (21.6118, 36.0572) -> (17.3322, 32.3579) centre (21.3216, 32.0677) ccw projected
  arc A12 (21.6118, 36.0572) -> (25.8914, 39.7565) centre (21.9019, 40.0466) ccw projected
  line L7 (25.8914, 39.7565) -> (27, 55) projected
  line L8 (27, 55) -> (27, 362.5) projected
  circle A13 centre (9, 160) radius 1.6 projected
  circle A14 centre (9, 260) radius 1.6 projected
  circle A15 centre (-9, 260) radius 1.6 projected
  circle A16 centre (-9, 160) radius 1.6 projected
  circle A17 centre (18, 160) radius 1.6 projected
  circle A18 centre (18, 260) radius 1.6 projected
  circle A19 centre (-18, 260) radius 1.6 projected
  circle A20 centre (-18, 160) radius 1.6 projected
  circle A21 centre (0, 362.5) radius 1.6 projected
  circle A22 centre (-18, 362.5) radius 1.6 projected
  circle A23 centre (9, 362.5) radius 1.6 projected
  circle A24 centre (18, 362.5) radius 1.6 projected
  circle A25 centre (-9, 362.5) radius 1.6 projected
  line L9 (10, 39) -> (10, 33) projected
  arc A26 (6, 29) -> (10, 33) centre (6, 33) ccw projected
  line L10 (6, 29) -> (-6, 29) projected
  arc A27 (-10, 33) -> (-6, 29) centre (-6, 33) ccw projected
  line L11 (-10, 33) -> (-10, 39) projected
  arc A28 (-6, 43) -> (-10, 39) centre (-6, 39) ccw projected
  line L12 (-6, 43) -> (6, 43) projected
  arc A29 (10, 39) -> (6, 43) centre (6, 39) ccw projected
  circle A30 centre (0, 0) radius 13 projected
  circle A31 centre (18, 0) radius 1.6 projected
  circle A32 centre (-12, -12) radius 1.6 projected
  circle A33 centre (0, -18) radius 1.6 projected
  circle A34 centre (12, -12) radius 1.6 projected
  circle A35 centre (-18, 0) radius 1.6 projected
  circle A36 centre (-12, 12) radius 1.6 projected
  circle A37 centre (12, 12) radius 1.6 projected
  circle A38 centre (0, 18) radius 1.6 projected
  circle A39 centre (-9, 57.5) radius 1.6 projected
  circle A40 centre (-18, 57.5) radius 1.6 projected
  circle A41 centre (0, 57.5) radius 1.6 projected
  circle A42 centre (18, 57.5) radius 1.6 projected
  circle A43 centre (9, 57.5) radius 1.6 projected
extrude "돌출16" add sketch "스케치15" against normal blind 4 contours A21 | A22 | A23 | A24 | A25
sketch "스케치16" plane through (0, 0, 4) normal (0, 0, 1) x (1, 0, 0)
  circle A0 centre (0, 260) radius 1.6 projected
  circle A1 centre (0, 160) radius 1.6 projected
  arc A2 (27, 362.5) -> (23, 366.5) centre (23, 362.5) ccw projected
  line L0 (23, 366.5) -> (-23, 366.5) projected
  arc A3 (-23, 366.5) -> (-27, 362.5) centre (-23, 362.5) ccw projected
  line L1 (-27, 362.5) -> (-27, 55) projected
  line L2 (-27, 55) -> (-25.8914, 39.7565) projected
  arc A4 (-25.8914, 39.7565) -> (-21.6118, 36.0572) centre (-21.9019, 40.0466) ccw projected
  arc A5 (-17.3322, 32.3579) -> (-21.6118, 36.0572) centre (-21.3216, 32.0677) ccw projected
  line L3 (-17.3322, 32.3579) -> (-16.4617, 20.3895) projected
  arc A6 (-20.1611, 16.1099) -> (-16.4617, 20.3895) centre (-20.4512, 20.0993) ccw projected
  arc A7 (-20.1611, 16.1099) -> (-23.8604, 11.8303) centre (-19.8709, 12.1204) ccw projected
  line L4 (-23.8604, 11.8303) -> (-23, 0) projected
  arc A8 (-23, 0) -> (23, 0) centre (0, 0) ccw projected
  line L5 (23, 0) -> (23.8604, 11.8303) projected
  arc A9 (23.8604, 11.8303) -> (20.1611, 16.1099) centre (19.8709, 12.1204) ccw projected
  arc A10 (16.4617, 20.3895) -> (20.1611, 16.1099) centre (20.4512, 20.0993) ccw projected
  line L6 (16.4617, 20.3895) -> (17.3322, 32.3579) projected
  arc A11 (21.6118, 36.0572) -> (17.3322, 32.3579) centre (21.3216, 32.0677) ccw projected
  arc A12 (21.6118, 36.0572) -> (25.8914, 39.7565) centre (21.9019, 40.0466) ccw projected
  line L7 (25.8914, 39.7565) -> (27, 55) projected
  line L8 (27, 55) -> (27, 362.5) projected
  circle A13 centre (9, 160) radius 1.6 projected
  circle A14 centre (9, 260) radius 1.6 projected
  circle A15 centre (-9, 260) radius 1.6 projected
  circle A16 centre (-9, 160) radius 1.6 projected
  circle A17 centre (18, 160) radius 1.6 projected
  circle A18 centre (18, 260) radius 1.6 projected
  circle A19 centre (-18, 260) radius 1.6 projected
  circle A20 centre (-18, 160) radius 1.6 projected
  line L9 (10, 39) -> (10, 33) projected
  arc A21 (6, 29) -> (10, 33) centre (6, 33) ccw projected
  line L10 (6, 29) -> (-6, 29) projected
  arc A22 (-10, 33) -> (-6, 29) centre (-6, 33) ccw projected
  line L11 (-10, 33) -> (-10, 39) projected
  arc A23 (-6, 43) -> (-10, 39) centre (-6, 39) ccw projected
  line L12 (-6, 43) -> (6, 43) projected
  arc A24 (10, 39) -> (6, 43) centre (6, 39) ccw projected
  circle A25 centre (0, 0) radius 13 projected
  circle A26 centre (18, 0) radius 1.6 projected
  circle A27 centre (-12, -12) radius 1.6 projected
  circle A28 centre (0, -18) radius 1.6 projected
  circle A29 centre (12, -12) radius 1.6 projected
  circle A30 centre (-18, 0) radius 1.6 projected
  circle A31 centre (-12, 12) radius 1.6 projected
  circle A32 centre (12, 12) radius 1.6 projected
  circle A33 centre (0, 18) radius 1.6 projected
  circle A34 centre (-9, 57.5) radius 1.6 projected
  circle A35 centre (-18, 57.5) radius 1.6 projected
  circle A36 centre (0, 57.5) radius 1.6 projected
  circle A37 centre (18, 57.5) radius 1.6 projected
  circle A38 centre (9, 57.5) radius 1.6 projected
  circle A39 centre (-5, 362.5) radius 1.6
  circle A40 centre (17, 362.5) radius 1.6
  circle A41 centre (-17, 362.5) radius 1.6
  circle A42 centre (5, 362.5) radius 1.6
  dimension "d90" = 3.2
  dimension "d91" = 3.2
  dimension "d92" = 3.2
  dimension "d93" = 12
  dimension "d94" = 10
  dimension "d95" = 12
  dimension "d96" = 10
  constraints: 4 centre point
  measures "d90" diameter of A39
  measures "d91" diameter of A40
  measures "d92" diameter of A41
  measures "d93" distance of A41.centre A39.centre
  measures "d94" distance of A39.centre A42.centre
  measures "d95" distance of A42.centre A40.centre
  measures "d96" distance from line of L1 A41.centre
extrude "돌출17" cut sketch "스케치16" against normal blind 4 contours A39 | A40 | A41 | A42
extrude "돌출18" [suppressed]
chamfer "모따기2" distance 1.5 angle 45 10 edges at (16.4, 57.5, 0) (7.4, 57.5, 0) (-1.6, 57.5, 0) (-10.6, 57.5, 0) (-19.6, 57.5, 0) (16.4, 57.5, 4) (7.4, 57.5, 4) (-1.6, 57.5, 4) (-10.6, 57.5, 4) (-19.6, 57.5, 4)
fillet "모깎기7" [suppressed]
sketch "스케치19" plane through (0, 0, 4) normal (0, 0, 1) x (1, 0, 0)
  circle A0 centre (5, 362.5) radius 1.6 projected
  circle A1 centre (-5, 362.5) radius 1.6 projected
  circle A2 centre (17, 362.5) radius 1.6 projected
  circle A3 centre (-17, 362.5) radius 1.6 projected
  circle A4 centre (0, 260) radius 1.6 projected
  circle A5 centre (0, 160) radius 1.6 projected
  arc A6 (27, 362.5) -> (23, 366.5) centre (23, 362.5) ccw projected
  line L0 (23, 366.5) -> (-23, 366.5) projected
  arc A7 (-23, 366.5) -> (-27, 362.5) centre (-23, 362.5) ccw projected
  line L1 (-27, 362.5) -> (-27, 55) projected
  line L2 (-27, 55) -> (-25.8914, 39.7565) projected
  arc A8 (-25.8914, 39.7565) -> (-21.6118, 36.0572) centre (-21.9019, 40.0466) ccw projected
  arc A9 (-17.3322, 32.3579) -> (-21.6118, 36.0572) centre (-21.3216, 32.0677) ccw projected
  line L3 (-17.3322, 32.3579) -> (-16.4617, 20.3895) projected
  arc A10 (-20.1611, 16.1099) -> (-16.4617, 20.3895) centre (-20.4512, 20.0993) ccw projected
  arc A11 (-20.1611, 16.1099) -> (-23.8604, 11.8303) centre (-19.8709, 12.1204) ccw projected
  line L4 (-23.8604, 11.8303) -> (-23, 0) projected
  arc A12 (-23, 0) -> (23, 0) centre (0, 0) ccw projected
  line L5 (23, 0) -> (23.8604, 11.8303) projected
  arc A13 (23.8604, 11.8303) -> (20.1611, 16.1099) centre (19.8709, 12.1204) ccw projected
  arc A14 (16.4617, 20.3895) -> (20.1611, 16.1099) centre (20.4512, 20.0993) ccw projected
  line L6 (16.4617, 20.3895) -> (17.3322, 32.3579) projected
  arc A15 (21.6118, 36.0572) -> (17.3322, 32.3579) centre (21.3216, 32.0677) ccw projected
  arc A16 (21.6118, 36.0572) -> (25.8914, 39.7565) centre (21.9019, 40.0466) ccw projected
  line L7 (25.8914, 39.7565) -> (27, 55) projected
  line L8 (27, 55) -> (27, 362.5) projected
  circle A17 centre (9, 160) radius 1.6 projected
  circle A18 centre (9, 260) radius 1.6 projected
  circle A19 centre (-9, 260) radius 1.6 projected
  circle A20 centre (-9, 160) radius 1.6 projected
  circle A21 centre (18, 160) radius 1.6 projected
  circle A22 centre (18, 260) radius 1.6 projected
  circle A23 centre (-18, 260) radius 1.6 projected
  circle A24 centre (-18, 160) radius 1.6 projected
  line L9 (10, 39) -> (10, 33) projected
  arc A25 (6, 29) -> (10, 33) centre (6, 33) ccw projected
  line L10 (6, 29) -> (-6, 29) projected
  arc A26 (-10, 33) -> (-6, 29) centre (-6, 33) ccw projected
  line L11 (-10, 33) -> (-10, 39) projected
  arc A27 (-6, 43) -> (-10, 39) centre (-6, 39) ccw projected
  line L12 (-6, 43) -> (6, 43) projected
  arc A28 (10, 39) -> (6, 43) centre (6, 39) ccw projected
  circle A29 centre (0, 0) radius 13 projected
  circle A30 centre (18, 0) radius 1.6 projected
  circle A31 centre (-12, -12) radius 1.6 projected
  circle A32 centre (0, -18) radius 1.6 projected
  circle A33 centre (12, -12) radius 1.6 projected
  circle A34 centre (-18, 0) radius 1.6 projected
  circle A35 centre (-12, 12) radius 1.6 projected
  circle A36 centre (12, 12) radius 1.6 projected
  circle A37 centre (0, 18) radius 1.6 projected
  line L13 (0, 129.9632) -> (-21.2132, 108.75)
  line L14 (0, 129.9632) -> (30, 129.9632) construction
  line L15 (-21.2132, 108.75) -> (0, 87.5368)
  line L16 (0, 87.5368) -> (0, 129.9632)
  line L17 (0, 129.9632) -> (23.2108, 129.9632) construction
  line L18 (-21.2132, 108.75) -> (10.7868, 108.75)
  line L19 (0, 129.9632) -> (10.7868, 108.75)
  line L20 (10.7868, 108.75) -> (0, 87.5368)
  arc A38 (10.7868, 108.75) -> (0, 129.9632) centre (4.0092, 118.6528) ccw
  arc A39 (0, 87.5368) -> (10.7868, 108.75) centre (4.0092, 98.8472) ccw
  line L21 (0, 332.4632) -> (-21.2132, 311.25)
  line L22 (0, 332.4632) -> (30, 332.4632) construction
  line L23 (-21.2132, 311.25) -> (0, 290.0368)
  line L24 (0, 290.0368) -> (0, 332.4632)
  line L25 (0, 332.4632) -> (23.2108, 332.4632) construction
  line L26 (-21.2132, 311.25) -> (10.7868, 311.25)
  line L27 (0, 332.4632) -> (10.7868, 311.25)
  line L28 (10.7868, 311.25) -> (0, 290.0368)
  arc A40 (10.7868, 311.25) -> (0, 332.4632) centre (4.0092, 321.1528) ccw
  arc A41 (0, 290.0368) -> (10.7868, 311.25) centre (4.0092, 301.3472) ccw
  line L29 (0, 366.5) -> (0, 0) construction
  line L30 (0, 362.5) -> (0, 260)
  circle A42 centre (0, 260) radius 1.6 projected
  circle A43 centre (0, 160) radius 1.6 projected
  line L31 (0, 260) -> (0, 160)
  circle A44 centre (0, 57.5) radius 1.6 projected
  line L32 (0, 160) -> (0, 57.5)
  line L33 (0, 231.2132) -> (-21.2132, 210)
  line L34 (0, 231.2132) -> (30, 231.2132) construction
  line L35 (-21.2132, 210) -> (0, 188.7868)
  line L36 (0, 188.7868) -> (0, 231.2132)
  line L37 (0, 231.2132) -> (23.2108, 231.2132) construction
  line L38 (-21.2132, 210) -> (10.7868, 210)
  line L39 (0, 231.2132) -> (10.7868, 210)
  line L40 (10.7868, 210) -> (0, 188.7868)
  arc A45 (10.7868, 210) -> (0, 231.2132) centre (4.0092, 219.9028) ccw
  arc A46 (0, 188.7868) -> (10.7868, 210) centre (4.0092, 200.0972) ccw
  point P0 (0, 311.25)
  point P1 (0, 311.25)
  point P2 (0, 108.75)
  point P3 (0, 210)
  point P4 (0, 108.75)
  point P5 (0, 210)
  dimension "d122" = 30
  dimension "d123" = 135
  dimension "d124" = 30
  dimension "d127" = 32
  dimension "d128" = 12
  dimension "d130" = 12
  dimension "d131" = 30
  dimension "d132" = 135
  dimension "d133" = 30
  dimension "d134" = 32
  dimension "d135" = 12
  dimension "d136" = 12
  dimension "d137" = 30
  dimension "d138" = 135
  dimension "d139" = 30
  dimension "d140" = 32
  dimension "d141" = 12
  dimension "d142" = 12
  constraints: 56 end point, 12 point on circle, 7 midpoint, 6 centre point, 6 horizontal, 6 perpendicular, 4 point on line, 3 equal length, 2 collinear, 2 vertical
  measures "d122" distance of L13.start L13.end
  measures "d123" angle of L13 L14
  measures "d124" distance of L13.end L15.end
  measures "d127" distance of L13.end L18.end
  measures "d128" radius of A38
  measures "d130" radius of A39
  measures "d131" distance of L21.start L23.start
  measures "d132" angle of L21 L22
  measures "d133" distance of L23.start L23.end
  measures "d134" distance of L23.start L26.end
  measures "d135" radius of A40
  measures "d136" radius of A41
  measures "d137" distance of L33.start L33.end
  measures "d138" angle of L33 L34
  measures "d139" distance of L33.end L35.end
  measures "d140" distance of L33.end L38.end
  measures "d141" radius of A45
  measures "d142" radius of A46
extrude "돌출20" cut sketch "스케치19" against normal blind 4 contours A38 L19 | L19 L18 L16 | L16 L18 L13 | A45 L39 | L39 L38 L31 | L31 L38 L33 | L23 L26 L24 | L24 L26 L28 | L28 A41 | L21 L24 L26 | L24 L27 L26 | L27 A40 | L38 L40 L31 | L31 L35 L38 | A46 L40 | L18 L16 L15 | L18 L20 L16 | A39 L20
fillet "모깎기9" radius 10 6 edges at (0, 332.4632, 2) (0, 290.0368, 2) (0, 188.7868, 2) (0, 87.5368, 2) (0, 231.2132, 2) (0, 129.9632, 2)
fillet "모깎기10" radius 4 3 edges at (-21.2132, 311.25, 2) (-21.2132, 210, 2) (-21.2132, 108.75, 2)
equation "\"d4\" = 0.5 * d2"
